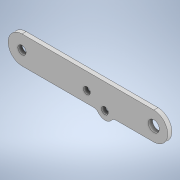
# Autodesk Inventor part: ramie_napinacza
Saved by Autodesk Inventor 2020.3 (Build 243373000, 373)
## iProperties
Created: 2021-10-24
Part Number: ramie_napinacza
Material: Ogólny
Document SubType Name: Modeling
Designer: patry
Density: 1 g/cm^3
Appearance: Domyślna
Author: patry
Autodesk Inventor part; units mm, degrees
ref_plane "YZ Plane" through (0, 0, 0) normal (1, 0, 0) x (0, 1, 0)
ref_plane "XZ Plane" through (0, 0, 0) normal (0, 1, 0) x (-1, 0, 0)
ref_plane "XY Plane" through (0, 0, 0) normal (0, 0, 1) x (1, 0, 0)
sketch "Szkic1" plane through (0, 0, 0) normal (0, 0, 1) x (1, 0, 0)
  line L0 (0, 0) -> (95, 0) construction
  line L1 (0, -10) -> (5.8348, -10)
  line L2 (95, 10) -> (0, 10)
  arc A0 (0, 10) -> (0, -10) centre (0, 0) ccw
  arc A1 (95, -10) -> (95, 10) centre (95, 0) ccw
  line L3 (5.8348, -10) -> (51.7624, -10)
  arc A2 (54.9624, -11.6) -> (64.5624, -11.6) centre (59.7624, -8) ccw
  line L4 (67.7624, -10) -> (95, -10)
  arc A3 (54.9624, -11.6) -> (51.7624, -10) centre (51.7624, -14) ccw
  arc A4 (67.7624, -10) -> (64.5624, -11.6) centre (67.7624, -14) ccw
  point P0 (47.5, 0)
  point P1 (46.7624, -2)
  point P2 (65.4193, -10)
  point P3 (54.1056, -10)
  point P4 (54.7624, -1)
  dimension "d0" = 95
  dimension "d1" = 20
  dimension "d23" = 12
  dimension "d24" = 4
  dimension "d34" = 8
  dimension "d35" = 5
  dimension "d36" = 7
  dimension "d37" = 1
  dimension "d38" = 6
  dimension "d40" = 40.25
  dimension "d41" = 1
  constraints: 12 end point, 12 point on circle, 12 tangent, 5 centre point, 3 coincident, 3 parallel, 2 point on line, 1 equal radius, 1 horizontal, 1 midpoint
  measures "d0" distance of L0.start L0.end
  measures "d1" diameter of A1
  measures "d23" diameter of A2
  measures "d24" radius of A3
  measures "d34" horizontal distance of point (54.762, -1) point (46.762, -2)
  measures "d35" horizontal distance of A2.centre point (54.762, -1)
  measures "d36" vertical distance of A2.centre point (54.762, -1)
  measures "d37" vertical distance of point (46.762, -2) point (54.762, -1)
  measures "d38" vertical distance of point (59.762, -8) point (46.762, -2)
  measures "d40" distance of point (54.762, -1) point (95, 0)
  measures "d41" distance from line of point (54.762, -1) L0
extrude "Wyciągnięcie proste1" add sketch "Szkic1" along normal blind 3
hole "Otwór1" at (95, 0, 0) direction (0, 0, 1) diameter 8 end through all
hole "Otwór2" at (46.7624, -2, 0) at (59.7624, -8, 0) direction (0, 0, 1) diameter 5 end through all
hole "Otwór3" at (0, 0, 0) direction (0, 0, 1) diameter 6 end through all
